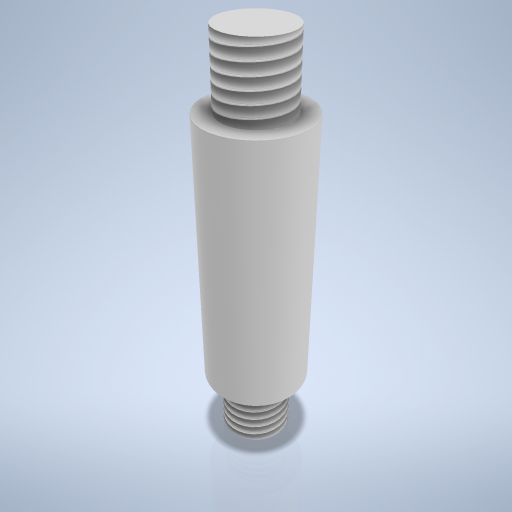
# Autodesk Inventor part: 17
Saved by Autodesk Inventor 2024.2 (Build 282272000, 272)
## iProperties
Created: 2024-05-05
Part Number: 17
Material: Generisch
Document SubType Name: Modeling
Designer: Fabri
Density: 1 g/cm^3
Appearance: Vorgabe
Author: Fabri
Autodesk Inventor part; units mm, degrees
ref_plane "YZ Plane" through (0, 0, 0) normal (1, 0, 0) x (0, 1, 0)
ref_plane "XZ Plane" through (0, 0, 0) normal (0, 1, 0) x (-1, 0, 0)
ref_plane "XY Plane" through (0, 0, 0) normal (0, 0, 1) x (1, 0, 0)
sketch "Skizze1" plane through (0, 0, 0) normal (0, 1, 0) x (-1, 0, 0)
  line L0 (0, 0) -> (4, 0)
  line L1 (4, 0) -> (4, -8)
  line L2 (4, -8) -> (6, -8)
  line L3 (6, -8) -> (6, -40)
  line L4 (6, -40) -> (4, -40)
  line L5 (4, -40) -> (4, -48)
  line L6 (4, -48) -> (0, -48)
  line L7 (0, -48) -> (0, 0)
  dimension "d0" = 8
  dimension "d1" = 32
  dimension "d2" = 8
  dimension "d3" = 8
  dimension "d4" = 12
  constraints: 16 end point, 6 perpendicular, 2 point on line, 1 horizontal
  measures "d0" distance between parallel lines of L2 L0
  measures "d1" distance of L2.end L3.end
  measures "d2" distance between parallel lines of L6 L4
  measures "d3" diameter of L1 L7
  measures "d4" diameter of L3 L7
revolve "Umdrehung1" add sketch "Skizze1" angle 360 about axis through (0, 0, -48) along (0, 0, 1)
thread "Gewinde1" size "M8x1.25" class "6g" standard "ISO Metric profile" full length
equation "\"d2\" = d0"
